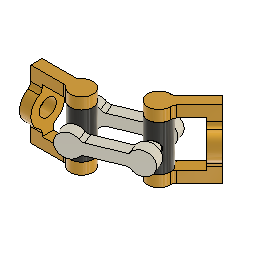
Cardan Joint v1 (Autodesk Fusion 360 design; units mm, degrees)
Autodesk Fusion 360 part; units mm, degrees
note: some values were not read from the file. Chosen so that the rebuilt part matches the saved one: which bodies a step acts on. Set by a fixed rule: which sketch regions a step uses.
sketch "Sketch1" plane through (0, 0, 0) normal (0, 1, 0) x (1, 0, 0) in component "Yoke"
  line L0 (-20, 30) -> (20, 30)
  line L1 (20, -30) -> (-20, -30)
  line L2 (-20, -30) -> (-20, 30)
  line L3 (-10, 20) -> (10, 20)
  line L4 (10, -20) -> (-10, -20)
  line L5 (-10, -20) -> (-10, 20)
  line L6 (10, -20) -> (20, -20)
  line L7 (10, 20) -> (20, 20)
  line L8 (20, 30) -> (20, 20)
  line L9 (20, -20) -> (20, -30)
  dimension "d1" = 40
  dimension "d2" = 60
  constraint horizontal L0
  constraint perpendicular L0 L8
  constraint parallel L0 L1
  constraint parallel L2 L8
  constraint coincident L6.end L8
  constraint perpendicular L6 L8
  constraint perpendicular L7 L8
  constraint collinear L8 L9
  measures "d1" distance of L1.start L1.end
  measures "d2" distance of L0.end L1.start
extrude "Extrude1" add sketch "Sketch1" along normal mid plane 10 makes body 1 in component "Yoke"
sketch "Sketch2" plane through (-10, 0, 0) normal (1, 0, 0) x (0, 1, 0) in component "Yoke"
  line L0 (-5, -20) -> (5, -20)
  line L1 (5, -20) -> (5, 20)
  line L2 (5, 20) -> (-5, 20)
  line L3 (-5, 20) -> (-5, -20)
  circle A0 centre (0, 0) radius 7.5
  circle A1 centre (0, 0) radius 15
  dimension "d6" = 15
  dimension "d7" = 30
  constraint coincident A0.centre A1.centre
  measures "d6" diameter of A0
  measures "d7" diameter of A1
extrude "Extrude2" cut sketch "Sketch2" against normal blind 32 contours L1 L3 A0 bodies 1 makes body 2 at (-3.3333, -5, -26.6667) in component "Yoke"
extrude "Extrude3" add sketch "Sketch2" against normal blind 10 contours L3 A0 A1 | L1 L3 A0 A1 | L1 A0 A1 | L1 L3 A0 A1 bodies 1 2 in component "Yoke"
cylinder "CylinderPrimitive1" add diameter 20 height -10 placed x (0, 1, 0) y (1, 0, 0) z (0, 0, -1) at (20, 0, 20) bodies 1 in component "Yoke"
cylinder "CylinderPrimitive2" add diameter 10 height 5 placed x (0, 1, 0) y (1, 0, 0) z (0, 0, -1) at (20, 0, 20) bodies 1 in component "Yoke"
fillet "Fillet1" radius 5 4 edges at (-15, -5, -14.1421) (-15, -5, 14.1421) (-15, 5, -14.1421) (-15, 5, 14.1421) on bodies 1 in component "Yoke"
fillet "Fillet2" radius 5 2 edges at (11.3397, -5, 25) (11.3397, 5, 25) on bodies 1 in component "Yoke"
fillet "Fillet3" radius 0.5 2 edges at (18.1919, -4.6616, 15) (21.8081, -4.6616, 20) on bodies 1 in component "Yoke"
mirror "Mirror1" about plane through (0, 0, 0) normal (0, 0, 1) of "CylinderPrimitive1", "CylinderPrimitive2", "Fillet2", "Fillet3" in component "Yoke"
cylinder "CylinderPrimitive1'" add diameter 20 height 40 placed x (1, 0, 0) y (0, 1, 0) z (0, 0, 1) at (20, 0, -20) separate body makes body 3 in component "Pin"
hole "Hole1" at (20, -10, 0) direction (0, 1, 0) diameter 10 end through all bodies 3 in component "Pin"
combine "Combine1" operation cut target body 3 tool bodies 1 keep tools in component "Pin"
fillet "Fillet1'" radius 0.5 3 edges at (25, -8.6603, 0) (15, -8.6603, 0) (25, 8.6603, 0) on bodies 3 in component "Pin"
sketch "Sketch1 (2)" plane through (0, 0, 0) normal (0, 1, 0) x (1, 0, 0) in component "Center Block"
  line L0 (30, -20) -> (12.5464, -20)
  circle A0 centre (20, 0) radius 5
  circle A1 centre (20, 0) radius 10
  dimension "d32" = 10
  dimension "d33" = 20
  dimension "d34" = 20
  dimension "d35" = 10
  constraint concentric A0 A1
  measures "d32" diameter of A0
  measures "d33" diameter of A1
  measures "d34" vertical distance of L0.start A0.centre
  measures "d35" horizontal distance of L0.start A0.centre
extrude "Extrude1'" add sketch "Sketch1 (2)" along normal mid plane 25 separate body contours A0 makes body 4 in component "Center Block"
extrude "Extrude2'" add sketch "Sketch1 (2)" against normal blind 10 from surface at -12.5 contours A0 | A1 bodies 4 in component "Center Block"
extrude "Extrude3'" add sketch "Sketch1 (2)" along normal blind 10 from surface at 12.5 contours A0 | A1 bodies 4 in component "Center Block"
copy_body "CopyPasteBodies1" bodies 4 makes body 5 in component "Center Block"
move_body "Move1" bodies 5 to x (1, 0, 0) y (0, 1, 0) z (0, 0, 1) at (50, 0, 0) in component "Center Block"
sketch "Sketch2 (2)" plane through (0, -22.5, 0) normal (0, -1, 0) x (1, 0, 0) in component "Center Block"
  circle A0 centre (70, 0) radius 10
  line L0 (20, 5) -> (70, 5)
  line L1 (70, 5) -> (70, -5)
  line L2 (70, -5) -> (20, -5)
  line L3 (20, -5) -> (20, 5)
  circle A1 centre (20, 0) radius 10
  dimension "d44" = 50
  dimension "d45" = 10
  dimension "d46" = 5
  constraint horizontal L0
  constraint vertical L1
  constraint horizontal L2
  constraint vertical L3
  measures "d44" distance of L0.start L0.end
  measures "d45" distance of L0.start L2.end
  measures "d46" distance of L0 A1.centre
extrude "Extrude4" add sketch "Sketch2 (2)" against normal blind 10 contours A0 L0 L2 A1 bodies 4 5 in component "Center Block"
mirror "Mirror1'" about plane through (0, 0, 0) normal (0, 1, 0) of "Extrude4" in component "Center Block"
fillet "Fillet1''" radius 5 7 edges at (28.6603, -17.5, 5) (28.6603, 17.5, 5) (61.3397, -17.5, 5) (61.3397, 17.5, 5) (28.6603, -17.5, -5) (61.3397, -17.5, -5) (28.6603, 17.5, -5) on bodies 4 in component "Center Block"
cylinder "CylinderPrimitive1''" add diameter 15 height 50 placed x (0, 0, 1) y (0, 1, 0) z (-1, 0, 0) at (-20, 0, 0) separate body makes body 6 in component "Component"
component "Yoke" placed x (1, 0, 0) y (0, 1, 0) z (0, 0, 1) at (-10, 0, 0)
component "Yoke" placed x (-0.707107, -0.707107, 0) y (0.707107, -0.707107, 0) z (0, 0, 1) at (68.0543, 38.7852, 0)
component "Pin" placed x (0.92388, 0.382683, 0) y (-0.382683, 0.92388, 0) z (0, 0, 1) at (-8.4776, -7.6537, 0)
component "Pin" placed x (0.92388, 0.382683, 0) y (0.382683, -0.92388, 0) z (0, 0, -1) at (35.4345, 16.9894, 0)
component "Center Block" placed x (0.92388, 0.382683, 0) y (0.382683, -0.92388, 0) z (0, 0, -1) at (-8.6618, -7.2089, 0)
component "Component" placed x (1, 0, 0) y (0, 1, 0) z (0, 0, 1) at (0, 0, 0)
component "Component" placed x (0.707107, 0.707107, 0) y (-0.707107, 0.707107, 0) z (0, 0, 1) at (124.6228, 95.3537, 0)
